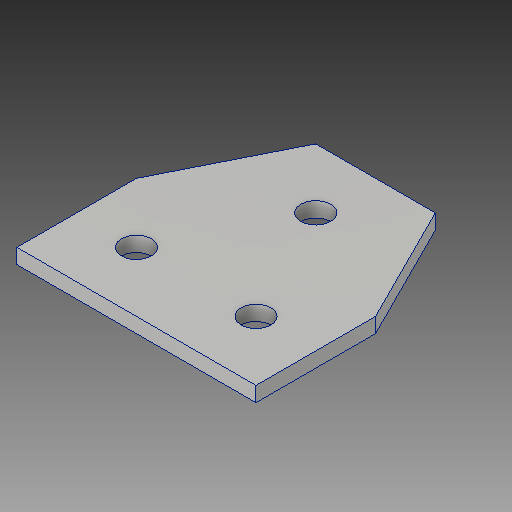
# Autodesk Inventor part: 15102898-16-P-0212
Saved by Autodesk Inventor 2017 (Build 210142000, 142)
## iProperties
Created: 2016-10-05
Part Number: 15102898-16-P-0212
Material: Aluminum 6061
Document SubType Name: Modeling
Designer: gus
Density: 2.7 g/cm^3
Appearance: Aluminum - Flat
Mass: 18.5428 g
Surface Area: 50.9967 cm^2
Volume: 6.86769 cm^3
Author: gus
Autodesk Inventor part; units mm, degrees
ref_plane "YZ Plane" through (0, 0, 0) normal (1, 0, 0) x (0, 1, 0)
ref_plane "XZ Plane" through (0, 0, 0) normal (0, 1, 0) x (-1, 0, 0)
ref_plane "XY Plane" through (0, 0, 0) normal (0, 0, 1) x (1, 0, 0)
sketch "Sketch1" plane through (0, 0, 0) normal (0, 1, 0) x (-1, 0, 0)
  line L0 (0, 0) -> (50.8, 0)
  line L1 (50.8, 0) -> (50.8, -25.4)
  line L2 (50.8, -25.4) -> (38.1, -50.8)
  line L3 (38.1, -50.8) -> (12.7, -50.8)
  line L4 (12.7, -50.8) -> (0, -25.4)
  line L5 (0, -25.4) -> (0, 0)
  circle A0 centre (12.7, -12.7) radius 3.175
  circle A1 centre (38.1, -12.7) radius 3.175
  circle A2 centre (25.4, -38.1) radius 3.175
  dimension "d0" = 25.4
  dimension "d1" = 50.8
  dimension "d2" = 25.4
  dimension "d3" = 50.8
  dimension "d4" = 12.7
  dimension "d5" = 6.35
  dimension "d6" = 6.35
  dimension "d7" = 12.7
  dimension "d8" = 12.7
  dimension "d9" = 12.7
  dimension "d10" = 12.7
  dimension "d11" = 6.35
  dimension "d12" = 12.7
  dimension "d13" = 12.7
  constraints: 12 end point, 3 centre point, 2 parallel, 1 equal length, 1 horizontal, 1 perpendicular
  measures "d0" distance of L0.end L1.end
  measures "d1" distance of L0.start L0.end
  measures "d2" distance of L2.end L3.end
  measures "d3" distance between parallel lines of L0 L3
  measures "d4" horizontal distance of L1.end L2.end
  measures "d5" diameter of A0
  measures "d6" diameter of A1
  measures "d7" distance from line of L1 A1.centre
  measures "d8" distance from line of L0 A1.centre
  measures "d9" distance from line of L5 A0.centre
  measures "d10" distance from line of L0 A0.centre
  measures "d11" diameter of A2
  measures "d12" distance from line of L3 A2.centre
  measures "d13" horizontal distance of A2.centre L3.end
extrude "Extrusion1" add sketch "Sketch1" along normal blind 3.175
body "Solid1"
